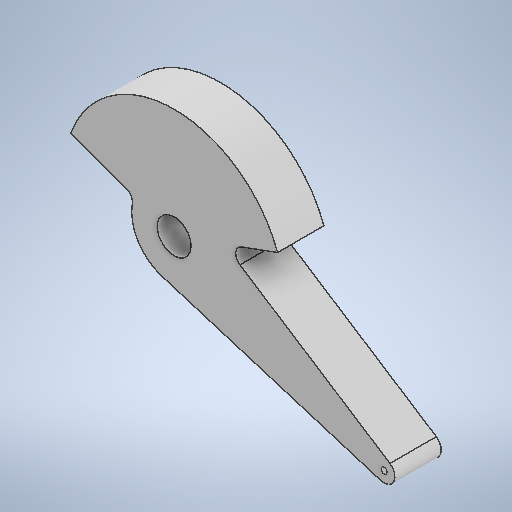
# Autodesk Inventor part: RT_ARM_MC_008_Capstand_Arm
Saved by Autodesk Inventor 2025.3 (Build 293356000, 356)
## iProperties
Created: 2026-07-28
Part Number: RT_ARM_MC_008_Capstand_Arm
Material: Generic
Document SubType Name: Modeling
Designer: louis
Density: 1 g/cm^3
Appearance: Default
Author: louis
Autodesk Inventor part; units mm, degrees
ref_plane "YZ Plane" through (0, 0, 0) normal (1, 0, 0) x (0, 1, 0)
ref_plane "XZ Plane" through (0, 0, 0) normal (0, 1, 0) x (-1, 0, 0)
ref_plane "XY Plane" through (0, 0, 0) normal (0, 0, 1) x (1, 0, 0)
sketch "Sketch1" plane through (0, 0, 0) normal (0, 0, 1) x (1, 0, 0)
  circle A0 centre (0, 0) radius 11
  circle A1 centre (0, 84) radius 14 construction
  circle A2 centre (0, 0) radius 72 construction
  circle A3 centre (0, 84) radius 12 construction
  line L0 (0, 84) -> (0, 0) construction
  line L1 (-67.6579, 24.6255) -> (0, 0) construction
  line L2 (67.6579, 24.6255) -> (0, 0) construction
  circle A4 centre (0, 84) radius 35 construction
  line L3 (-60, 71.9226) -> (-60, 144) construction
  line L4 (-60, 144) -> (60, 144) construction
  line L5 (60, 144) -> (60, 71.9226) construction
  circle A5 centre (0, 0) radius 27.5
  line L6 (25.3583, -10.6399) -> (60, 71.9226) construction
  line L7 (-60, 71.9226) -> (-25.3583, -10.6399) construction
  line L8 (0, 0) -> (135.9462, -63.3927) construction
  line L9 (-24.7487, 59.2513) -> (24.7487, 59.2513) construction
  circle A6 centre (0, 84) radius 60 construction
  arc A7 (67.6579, 24.6255) -> (-67.6579, 24.6255) centre (0, 0) ccw
  arc A8 (66.9531, 24.3689) -> (-66.9531, 24.3689) centre (0, 0) ccw
  line L10 (67.3977, 25.3289) -> (67.4014, 25.3302)
  circle A9 centre (135.9462, -63.3927) radius 2
  circle A10 centre (135.9462, -63.3927) radius 7
  line L11 (-67.6579, 24.6255) -> (0, 0)
  line L12 (0, 0) -> (67.6579, 24.6255)
  line L13 (-8.1067, -26.2779) -> (133.8826, -70.0817)
  line L14 (139.7438, -57.5124) -> (14.9192, 23.1013)
  point P0 (24.7487, 108.7487)
  point P1 (-24.7487, 108.7487)
  point P2 (-25.8415, 9.4056)
  point P3 (32.419, 11.7996)
  point P4 (66.9531, 24.3689)
  point P5 (-66.9531, 24.3689)
  dimension "d7" = 70
  dimension "d2" = 24
  dimension "d3" = 144
  dimension "d4" = 28
  dimension "d5" = 22
  dimension "d6" = 220
  dimension "d8" = 360
  dimension "d9" = 55
  dimension "d10" = 150
  dimension "d11" = 45
  dimension "d12" = 120
  dimension "d13" = 0.75
  dimension "d14" = 4
  dimension "d15" = 14
  constraints: 30 end point, 13 point on circle, 10 centre point, 10 coincident, 10 tangent, 2 collinear, 2 perpendicular, 2 vertical, 1 concentric, 1 horizontal, 1 point on line, 10 other
  measures "d2" diameter of A3
  measures "d3" diameter of A2
  measures "d4" diameter of A1
  measures "d5" diameter of A0
  measures "d9" diameter of A5
  measures "d10" distance of L8.start L8.end
  measures "d11" angle of L2 L8
  measures "d12" diameter of A6
  measures "d13" radial gap between concentric circles of A7 A8
  measures "d14" diameter of A9
  measures "d15" diameter of A10
extrude "Extrusion1" add sketch "Sketch1" along normal blind 30 contours A0 L12 A5 L11 | A0 L11 A5 L12 | L12 L14 A10 L13 A5 | A5 L14 L12 | L11 A8 L12 L14 A5 | A10
fillet "Fillet1" radius 6 2 edges at (-25.8415, 9.4056, 15) (32.419, 11.7996, 15)
equation "\"d3\" = 6 * d2"
body "Solid1"
